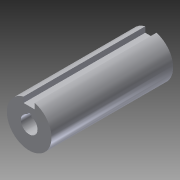
# Autodesk Inventor part: winch insert
Saved by Autodesk Inventor 2013 (Build 170138000, 138)
## iProperties
Created: 2013-02-06
Part Number: winch insert
Material: Aluminum 6061
Document SubType Name: Modeling
Designer: Arpan
Density: 1 g/cm^3
Author: Arpan
Autodesk Inventor part; units mm, degrees
ref_plane "YZ Plane" through (0, 0, 0) normal (1, 0, 0) x (0, 1, 0)
ref_plane "XZ Plane" through (0, 0, 0) normal (0, 1, 0) x (-1, 0, 0)
ref_plane "XY Plane" through (0, 0, 0) normal (0, 0, 1) x (1, 0, 0)
sketch "Sketch1" plane through (0, 0, 0) normal (0, 0, 1) x (1, 0, 0)
  circle A0 centre (0, 0) radius 12.7
  dimension "d0" = 25.4
  constraints: 1 centre point, 1 coincident
  measures "d0" diameter of A0
extrude "Extrusion1" add sketch "Sketch1" along normal blind 69.215
sketch "Sketch2" plane through (0, 0, 69.215) normal (0, 0, 1) x (1, 0, 0)
  circle A0 centre (0, 0) radius 12.7 projected
  line L0 (0, 0) -> (-3.6945, 0)
  line L1 (1.19, 5.802) -> (1.19, 4.6114)
  arc A1 (-1.19, 4.6114) -> (1.19, 4.6114) centre (0, 0) ccw
  line L2 (-1.19, 4.6114) -> (-1.1912, 4.6114)
  line L3 (-1.1912, 4.6114) -> (-1.1912, 5.802)
  line L4 (-1.1912, 5.802) -> (1.19, 5.802)
  constraints: 10 end point, 2 coincident, 2 point on circle, 1 centre point, 1 horizontal
extrude "Extrusion2" cut sketch "Sketch2" against normal blind 69.469 contours L1 A1 L3 L4
sketch "Sketch3" plane through (0, 0, 69.215) normal (0, 0, 1) x (1, 0, 0)
  line L0 (-1.1912, 4.6114) -> (-1.1912, 5.802) projected
  circle A0 centre (0, 0) radius 12.7 projected
  line L1 (0, 0) -> (-3.175, 0)
  line L2 (-3.175, 12.2967) -> (-3.175, 9.1217)
  line L3 (-3.175, 9.1217) -> (3.175, 9.1217)
  line L4 (3.175, 9.1217) -> (3.175, 12.2967)
  dimension "d5" = 3.175
  dimension "d6" = 3.175
  dimension "d7" = 6.35
  constraints: 8 end point, 3 perpendicular, 2 point on circle, 1 parallel
  measures "d5" distance of L1.start L1.end
  measures "d6" distance of L2.start L2.end
  measures "d7" distance of L2.end L3.end
extrude "Extrusion3" cut sketch "Sketch3" against normal blind 69.469 contours L4 L3 L2 A0 picked at (-0.3561, 10.2995)
body "Solid1"
